4mm (Autodesk Fusion 360 design; units mm, degrees)
Autodesk Fusion 360 part; units mm, degrees
note: some values were not read from the file. Chosen so that the rebuilt part matches the saved one: which bodies a step acts on. Set by a fixed rule: which sketch regions a step uses.
sketch "Sketch1" plane through (0, 0, 0) normal (0, 0, 1) x (1, 0, 0)
  line L0 (-28.9023, 0) -> (0, 0) construction
  line L1 (0, 0) -> (0, 16.228) construction
  line L2 (0, 16.228) -> (-28.9023, 16.228) construction
  line L3 (-28.9023, 16.228) -> (-28.9023, 0) construction
  dimension "d1" = 3
  text T0 "4 mm" font "Arial" height 3 align right bottom in box 28.9023 x 16.228 at (-28.9023, 0) x (1, 0) y (0, 1) spacing 1
  constraint coincident L0.end
extrude "Extrude1" add sketch "Sketch1" along normal blind 1 text T0 makes body 1 at (-2.822, 1.1003, 0) makes body 2 at (-6.3131, 1.1003, 0) makes body 3 at (-9.6978, 1.704, 0.3333)
sketch "Sketch2" plane through (0, 0, 0) normal (0, 0, 1) x (1, 0, 0)
  line L0 (-11.6828, 3.7332) -> (2.5, 3.7332)
  line L1 (2.5, 3.7332) -> (2.5, -2)
  line L2 (2.5, -2) -> (-11.6828, -2)
  line L3 (-11.6828, -2) -> (-11.6828, 3.7332)
  circle A0 centre (2.5, 0.8666) radius 2.8666
  circle A1 centre (-11.6828, 0.8666) radius 2.8666
  constraint horizontal L0
  constraint vertical L1
  constraint horizontal L2
  constraint vertical L3
  constraint coincident L1.end A0
  constraint tangent L2 A0
  constraint coincident L0.end A0
  constraint coincident L2.end A1
  constraint tangent L2 A1
  constraint coincident L0.start A1
extrude "Extrude2" add sketch "Sketch2" against normal blind 1 bodies 1 2 3
